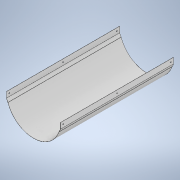
# Autodesk Inventor part: Ballslide
Saved by Autodesk Inventor 2022 (Build 260153000, 153)
## iProperties
Created: 2022-01-13
Part Number: Ballslide
Material: Generic
Document SubType Name: Modeling
Designer: tagaz
Density: 1 g/cm^3
Appearance: Default
Author: tagaz
Autodesk Inventor part; units mm, degrees
ref_plane "YZ Plane" through (0, 0, 0) normal (1, 0, 0) x (0, 1, 0)
ref_plane "XZ Plane" through (0, 0, 0) normal (0, 1, 0) x (-1, 0, 0)
ref_plane "XY Plane" through (0, 0, 0) normal (0, 0, 1) x (1, 0, 0)
sketch "Sketch1" plane through (0, 0, 0) normal (0, 0, 1) x (1, 0, 0)
  arc A0 (-114.2223, -38.8548) -> (0, -120.65) centre (0, 0) ccw
  line L0 (-120.65, 0) -> (-121.2596, 0)
  line L1 (120.65, 0) -> (121.2596, 0)
  line L2 (-121.2596, 0) -> (-121.2596, -25.4)
  line L3 (-120.65, 0) -> (-120.65, -25.4)
  line L4 (-121.2596, -25.4) -> (-120.65, -30.3117) construction
  line L5 (-120.65, -30.3117) -> (-117.4666, -33.4581) construction
  line L6 (-117.4666, -33.4581) -> (-114.5061, -39.9028) construction
  spline S0 degree 3 poles (-121.2596, -25.4) (-120.65, -30.3117) (-117.4666, -33.4581) (-114.5061, -39.9028) knots 1 1 1 1 2 2 2 2
  line L7 (-120.65, -25.4) -> (-120.1784, -29.1998) construction
  line L8 (-120.1784, -29.1998) -> (-116.9951, -32.3462) construction
  line L9 (-116.9951, -32.3462) -> (-114.2223, -38.8548) construction
  spline S1 degree 3 poles (-120.65, -25.4) (-120.1784, -29.1998) (-116.9951, -32.3462) (-114.2223, -38.8548) knots 1 1 1 1 2 2 2 2
  arc A1 (-114.5061, -39.9028) -> (0, -121.2596) centre (0, 0) ccw
  line L10 (0, 0) -> (0, -121.2596)
  arc A2 (0, -120.65) -> (114.2223, -38.8548) centre (0, 0) ccw
  line L11 (120.65, 0) -> (121.2596, 0)
  line L12 (121.2596, 0) -> (121.2596, -25.4)
  line L13 (120.65, 0) -> (120.65, -25.4)
  line L14 (121.2596, -25.4) -> (120.65, -30.3117) construction
  line L15 (120.65, -30.3117) -> (117.4666, -33.4581) construction
  line L16 (117.4666, -33.4581) -> (114.5061, -39.9028) construction
  spline S2 degree 3 poles (121.2596, -25.4) (120.65, -30.3117) (117.4666, -33.4581) (114.5061, -39.9028) knots 1 1 1 1 2 2 2 2
  spline S3 degree 3 poles (120.65, -25.4) (120.1784, -29.1998) (116.9951, -32.3462) (114.2223, -38.8548) knots 1 1 1 1 2 2 2 2
  line L17 (120.65, -25.4) -> (120.1784, -29.1998) construction
  line L18 (120.1784, -29.1998) -> (116.9951, -32.3462) construction
  line L19 (116.9951, -32.3462) -> (114.2223, -38.8548) construction
  arc A3 (0, -121.2596) -> (114.5061, -39.9028) centre (0, 0) ccw
  dimension "d0" = 241.3
  dimension "d1" = 0.6096
  dimension "d2" = 0.6096
  dimension "d5" = 25.4
  dimension "d6" = 25.4
  dimension "d7" = 1.1119
  dimension "d8" = 1.1119
  dimension "d9" = 3.1463
  dimension "d10" = 3.1833
  dimension "d11" = 0.6096
  dimension "d12" = 3.1833
  dimension "d14" = 14.5028
  dimension "d15" = 3.7998
  constraints: 16 end point, 8 point on circle, 8 symmetric about line, 4 centre point, 2 horizontal, 2 vertical, 1 coincident, 1 point on line, 1 tangent, 14 other
  measures "d0" diameter of A0
  measures "d1" distance of L0.start L0.end
  measures "d2" distance of L1.start L1.end
  measures "d5" distance of L0.end L2.end
  measures "d6" distance of L0.start L3.end
  measures "d7" vertical distance of L4.end L7.end
  measures "d8" vertical distance of L5.end L8.end
  measures "d9" vertical distance of L4.end L5.end
  measures "d10" horizontal distance of L7.end L8.end
  measures "d11" distance from line of L2 L4.end
  measures "d12" distance from line of L5.end L3
  measures "d14" vertical distance of L6.end L3.end
  measures "d15" vertical distance of L2.end L7.end
extrude "Extrusion1" add sketch "Sketch1" against normal blind 508
sketch "Sketch2" plane through (-120.65, -25.4, 0) normal (1, 0, 0) x (0, 0, -1)
  line L0 (0, 25.4) -> (0, 0) projected
  line L1 (0, 25.4) -> (508, 25.4) projected
  line L2 (508, 0) -> (508, 25.4) projected
  line L3 (0, 0) -> (508, 0) projected
  circle A0 centre (12.7, 12.7) radius 2.413
  circle A1 centre (254, 12.7) radius 2.413
  circle A2 centre (495.3, 12.7) radius 2.413
  dimension "d18" = 4.826
  dimension "d19" = 12.7
  dimension "d20" = 12.7
  dimension "d23" = 241.3
  constraints: 3 centre point, 1 horizontal, 4 other
  measures "d18" diameter of A0
  measures "d19" distance from line of L0 A0.centre
  measures "d20" distance from line of L1 A0.centre
  measures "d23" distance of A0.centre A1.centre
extrude "Extrusion2" cut sketch "Sketch2" along normal mid plane 560.3875 contours A0 | A1 | A2
body "Solid1"
